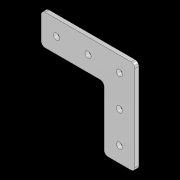
# Autodesk Inventor part: ConnectingPlatee
Saved by Autodesk Inventor 2022 (Build 260153000, 153)
## iProperties
Created: 2022-05-14
Part Number: ConnectingPlatee
Material: Generic
Document SubType Name: Modeling
Designer: tandu
Density: 1 g/cm^3
Appearance: Aluminum - Polished
Author: tandu
Autodesk Inventor part; units mm, degrees
ref_plane "YZ Plane" through (0, 0, 0) normal (1, 0, 0) x (0, 1, 0)
sketch "Sketch1" plane through (0, 0, 0) normal (0, 0, 1) x (1, 0, 0)
  line L0 (3.1494, 0) -> (-73.0506, 0)
  line L1 (-73.0506, 0) -> (-73.0506, -25.4)
  line L2 (-73.0506, -25.4) -> (-22.2506, -25.4)
  line L3 (3.1494, 0) -> (3.1494, -609.6) projected
  line L4 (-22.2506, -25.4) -> (-22.2506, -76.2)
  line L5 (-22.2506, -76.2) -> (3.1494, -76.2)
  line L6 (3.1494, 0) -> (3.1494, -76.2)
  line L7 (-73.0506, -12.7) -> (3.1494, -12.7) construction
  line L8 (-9.5506, -76.2) -> (-9.5506, 0) construction
  circle A0 centre (-60.3506, -12.7) radius 2.5082
  circle A1 centre (-9.5506, -63.5) radius 2.5083
  circle A2 centre (-34.9506, -12.7) radius 2.5083
  circle A3 centre (-9.5506, -12.7) radius 2.5083
  circle A4 centre (-9.5506, -38.1) radius 2.5083
  line L9 (-60.3506, -12.7) -> (-9.5506, -12.7) construction
  line L10 (-9.5506, -63.5) -> (-9.5506, -12.7) construction
  line L11 (-60.3506, -12.7) -> (-73.0506, -12.7) construction
  line L12 (-9.5506, -12.7) -> (-9.5506, 0) construction
  line L13 (-9.5506, -76.2) -> (-9.5506, -63.5) construction
  line L14 (-21.9966, -25.146) -> (-72.7966, -25.146)
  line L15 (-72.7966, -25.146) -> (-72.7966, -0.254)
  line L16 (-72.7966, -0.254) -> (2.8954, -0.254)
  line L17 (2.8954, -0.254) -> (2.8954, -75.946)
  line L18 (2.8954, -75.946) -> (-21.9966, -75.946)
  line L19 (-21.9966, -75.946) -> (-21.9966, -25.146)
  dimension "d0" = 76.2
  dimension "d1" = 25.4
  dimension "d4" = 5.0165
  dimension "d8" = 0.254
  constraints: 38 end point, 9 perpendicular, 5 centre point, 5 collinear, 5 midpoint, 5 point on line, 4 equal length, 4 equal radius, 1 horizontal, 1 vertical, 5 other
  measures "d0" distance of L0.start L0.end
  measures "d1" distance of L0.end L1.end
  measures "d4" diameter of A0
  measures "d8" distance between parallel lines of L2 L14
extrude "Extrusion1" add sketch "Sketch1" along normal blind 3.175 contours L14 L15 L16 L17 L18 L19
fillet "Fillet1" radius 3.175 6 edges at (-72.7966, -0.254, 1.5875) (-72.7966, -25.146, 1.5875) (-21.9966, -25.146, 1.5875) (2.8954, -0.254, 1.5875) (2.8954, -75.946, 1.5875) (-21.9966, -75.946, 1.5875)
ref_plane "Work Plane1" through (-69.6216, -12.7, 0) normal (0, 1, 0) x (1, 0, 0)
ref_plane "Work Plane2" through (-9.5506, -72.771, 0) normal (-1, 0, 0) x (0, 0, 1)
equation "\"d0\" = ConnectingPlateSize"
equation "\"d4\" = HoleSize"
equation "\"d8\" = Tolerance"
equation "\"d5\" = ConnectingPlateThickness"
equation "\"ConnectingPlateSize\" = 76.2"
equation "\"HoleSize\" = 5.0165"
equation "\"Tolerance\" = 0.254"
equation "\"ConnectingPlateThickness\" = 3.175"
body "Solid1"
